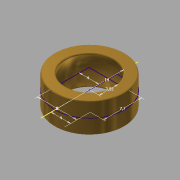
# Autodesk Inventor part: TULEJA
Saved by Autodesk Inventor 2013 (Build 170138000, 138)
## iProperties
Created: 2015-04-17
Part Number: TULEJA
Material: Brass, Soft Yellow
Document SubType Name: Modeling
Designer: Ultimate
Density: 1 g/cm^3
Author: Ultimate
Autodesk Inventor part; units mm, degrees
ref_plane "YZ Plane" through (0, 0, 0) normal (1, 0, 0) x (0, 1, 0)
ref_plane "XZ Plane" through (0, 0, 0) normal (0, 1, 0) x (-1, 0, 0)
ref_plane "XY Plane" through (0, 0, 0) normal (0, 0, 1) x (1, 0, 0)
sketch "Sketch1" plane through (0, 0, 0) normal (0, 0, 1) x (1, 0, 0)
  circle A0 centre (0, 0) radius 7
  line L0 (-4, 3.85) -> (4, 3.85)
  line L1 (4, 3.85) -> (4, -3.85)
  line L2 (4, -3.85) -> (-4, -3.85)
  line L3 (-4, -3.85) -> (-4, 3.85)
  arc A1 (0, -5.5518) -> (0, 5.5518) centre (0, 0) ccw
  line L4 (0, 5.5518) -> (0, -5.5518)
  line L5 (0, -9.8) -> (0, 9.8) projected
  dimension "d0" = 14
  dimension "d3" = 8
  dimension "d4" = 7.7
  dimension "d5" = 4
  dimension "d6" = 3.85
  dimension "d7" = 4
  constraints: 10 end point, 3 point on circle, 2 centre point, 2 coincident, 2 parallel, 2 perpendicular, 1 horizontal
  measures "d0" diameter of A0
  measures "d3" distance of L1.end L2.end
  measures "d4" distance of L0.end L1.end
  measures "d5" distance from line of point (0, 0) L3
  measures "d6" distance from line of L0 point (0, 0)
  measures "d7" distance between parallel lines of L4 L1
extrude "Extrusion1" add sketch "Sketch1" along normal mid plane 6
revolve "Revolution1" cut sketch "Sketch1" angle 360 about axis through (0, -10, 0) along (0, 1, 0) contours A1 L0 L4 | L4 L2 A1 | L1 L2 L4 L0 | A1 L1
fillet "Fillet1" radius 0.2 6 edges at (-7, 0, 3) (0, -4.6715, 3) (0, 4.6715, 3) (0, -4.6715, -3) (0, 4.6715, -3) (-7, 0, -3)
body "Solid1"
